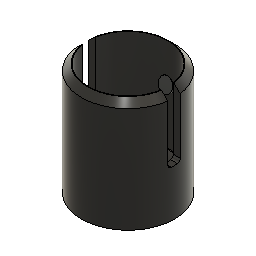
Endcap_switch_2023.04.26 (Autodesk Fusion 360 design; units mm, degrees)
Autodesk Fusion 360 part; units mm, degrees
sketch "Sketch1" plane through (0, 0, 0) normal (0, 1, 0) x (1, 0, 0)
  circle A0 centre (0, 0) radius 12.8
  circle A1 centre (0, 0) radius 10
  circle A2 centre (0, 0) radius 15
  dimension "d1" = 25.6
  dimension "d2" = 20
  dimension "d3" = 30
  constraint coincident A0.centre A1.centre
  measures "d1" diameter of A0
  measures "d2" diameter of A1
  measures "d3" diameter of A2
extrude "Extrude1" add sketch "Sketch1" along normal blind 30 contours A2 makes body 1
extrude "Extrude2" add sketch "Sketch1" against normal blind 6 contours A0 | A2 bodies 1
chamfer "Chamfer1" distance 2.5 distance2 1.5 1 edges at (-9.3233, 0, -3.6162) measured on face at (11.7818, 0, 1.1327) on bodies 1
ref_plane "WorkPlane1" through (0, 18, 0) normal (0, 1, 0) x (0, 0, 1)
sketch "Sketch3" plane through (0, 0, 0) normal (0, 0, 1) x (1, 0, 0)
  circle A0 centre (0, 18) radius 2.25
  point P0 (0, 18)
  dimension "d11" = 18
  dimension "d12" = 4.5
  constraint vertical origin A0.centre
  constraint coincident P0 A0.centre
  measures "d11" distance of origin A0.centre
  measures "d12" diameter of A0
extrude "Extrude3" add sketch "Sketch3" along normal mid plane 28 separate body makes body 2
ref_plane "WorkPlane2" through (-7.7034, 18, 0) normal (0, -0.258819, 0.965926) x (-1, 0, 0)
ref_plane "WorkPlane3" through (-7.7034, 14.9718, 11.3013) normal (0, -0.258819, 0.965926) x (-1, 0, 0)
split "Split1" by plane through (-7.7034, 14.9718, 11.3013) normal (0, -0.258819, 0.965926) bodies 2 makes body 3 at (-0.0106, 15.75, 13.17)
ref_plane "WorkPlane4" through (-7.7034, 18, 0) normal (0, 0.258819, 0.965926) x (-1, 0, 0)
ref_plane "WorkPlane5" through (-7.7034, 14.9718, -11.3013) normal (0, 0.258819, 0.965926) x (-1, 0, 0)
split "Split2" by plane through (-7.7034, 14.9718, -11.3013) normal (0, 0.258819, 0.965926) bodies 2 makes body 4 at (-0.0143, 20.25, 4.2385)
chamfer "Chamfer2" distance 2 distance2 2 1 edges at (-13.9849, 30, 5.4242) measured on face at (14.1632, 30, 1.3811) on bodies 1
sketch "Sketch4" plane through (0, 0, 0) normal (1, 0, 0) x (0, 0, -1)
  line L0 (-2, 30.7431) -> (2, 30.7431)
  line L1 (2, 30.7431) -> (2, 10)
  line L2 (1, 9) -> (-1, 9)
  line L3 (-2, 10) -> (-2, 30.7431)
  arc A0 (-2, 10) -> (-1, 9) centre (-1, 10) ccw
  arc A1 (1, 9) -> (2, 10) centre (1, 10) ccw
  point P0 (0, 30.7431)
  dimension "d23" = 4
  dimension "d24" = 1
  dimension "d25" = 1
  constraint horizontal L0
  constraint vertical L1
  constraint horizontal L2
  constraint vertical L3
  constraint midpoint L0 P0
  constraint vertical origin P0
  constraint tangent L2 A0
  constraint tangent L3 A0
  constraint tangent L1 A1
  constraint tangent L2 A1
  measures "d23" distance of L0.start L0.end
  measures "d24" radius of A0
  measures "d25" radius of A1
extrude "Extrude4" cut sketch "Sketch4" along normal mid plane 30 bodies 1
combine "Combine1" operation add target body 1 tool bodies 2 3
hidden bodies 4
